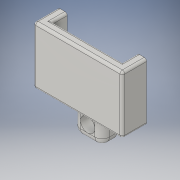
# Autodesk Inventor part: soporte esp1
Saved by Autodesk Inventor 2016 (Build 200138000, 138)
## iProperties
Created: 2017-03-11
Part Number: soporte esp1
Material: Generic
Document SubType Name: Modeling
Designer: jorge
Density: 1 g/cm^3
Appearance: White
Author: jorge
Autodesk Inventor part; units mm, degrees
ref_plane "YZ Plane" through (0, 0, 0) normal (1, 0, 0) x (0, 1, 0)
ref_plane "XZ Plane" through (0, 0, 0) normal (0, 1, 0) x (-1, 0, 0)
sketch "Sketch1" plane through (0, 0, 0) normal (0, 0, 1) x (1, 0, 0)
  line L0 (-32.1046, 28.3811) -> (-17.6046, 28.3811) projected
  line L1 (-32.1046, 3.3811) -> (-32.1046, 28.3811) projected
  line L2 (-17.6046, 3.3811) -> (-32.1046, 3.3811) projected
  line L3 (-17.6046, 28.3811) -> (-17.6046, 3.3811) projected
  circle A0 centre (-21.0446, 24.002) radius 0.51 projected
  circle A1 centre (-21.0446, 26.542) radius 0.51 projected
  circle A2 centre (-23.5846, 26.542) radius 0.51 projected
  circle A3 centre (-23.5846, 24.002) radius 0.51 projected
  circle A4 centre (-26.1246, 26.542) radius 0.51 projected
  circle A5 centre (-26.1246, 24.002) radius 0.51 projected
  circle A6 centre (-28.6646, 26.542) radius 0.51 projected
  circle A7 centre (-28.6646, 24.002) radius 0.51 projected
  line L4 (-17.6046, 3.3811) -> (-17.6046, 13.3811)
  line L5 (-17.6046, 13.3811) -> (-15.6046, 13.3811)
  line L6 (-15.6046, 13.3811) -> (-15.6046, 1.3811)
  line L7 (-15.6046, 1.3811) -> (-32.1046, 1.3811)
  line L8 (-32.1046, 1.3811) -> (-34.1046, 1.3811)
  line L9 (-34.1046, 1.3811) -> (-34.1046, 13.3811)
  line L10 (-34.1046, 13.3811) -> (-32.1046, 13.3811)
  point P0 (0, 0)
  dimension "d0" = 10
  dimension "d1" = 2
  dimension "d2" = 90
  dimension "d3" = 12
  dimension "d4" = 90
  dimension "d5" = 2
  dimension "d6" = 12
  constraints: 14 end point, 5 point on line, 2 perpendicular
  measures "d0" distance of L2.start L4.end
  measures "d1" distance of L4.end L5.end
  measures "d2" angle of L4 L5
  measures "d3" distance of L5.end L6.end
  measures "d4" angle of L6 L7
  measures "d5" distance of L7.end L8.end
  measures "d6" distance of L8.end L9.end
ref_plane "Work Plane1" through (-32.1046, 3.3811, 3.05) normal (0, 0, 1) x (1, 0, 0)
extrude "Extrusion1" add sketch "Sketch1" along normal up to surface (3.05 mm away) contours L1 L2 L3 L5 L6 L7 L8 L9 L10
sketch "Sketch2" plane through (-34.1046, 1.3811, 3.05) normal (0, 0, 1) x (1, 0, 0)
  line L0 (16.5, 12) -> (18.5, 12) projected
  line L1 (18.5, 12) -> (0, 12)
  line L2 (0, 12) -> (0, 0)
  line L3 (0, 0) -> (18.5, 0)
  line L4 (18.5, 0) -> (18.5, 12)
  point P0 (34.1046, -1.3811)
  constraints: 8 end point, 2 parallel, 1 horizontal, 1 perpendicular
extrude "Extrusion2" add sketch "Sketch2" along normal blind 2
sketch "Sketch3" plane through (-34.1046, 1.3811, 0) normal (0, -1, 0) x (1, 0, 0)
  line L0 (16.5, 0) -> (2, 0) projected
  line L1 (9.25, 0) -> (6.25, 0)
  line L2 (6.25, 0) -> (6.25, 3)
  line L3 (6.25, 3) -> (9.25, 3)
  line L4 (9.25, 3) -> (9.25, 0)
  line L5 (9.25, 3) -> (12.25, 3)
  line L6 (12.25, 3) -> (12.25, 0)
  line L7 (12.25, 0) -> (9.25, 0)
  line L8 (9.25, 0) -> (9.25, 3)
  point P0 (34.1046, 0)
  dimension "d11" = 3
  dimension "d12" = 3
  dimension "d13" = 3
  constraints: 16 end point, 4 parallel, 2 horizontal, 2 perpendicular, 1 midpoint, 1 point on line
  measures "d11" distance of L2.end L3.end
  measures "d12" distance of L1.end L2.end
  measures "d13" distance of L6.end L7.end
extrude "Extrusion3" add sketch "Sketch3" along normal blind 6
fillet "Fillet1" radius 1.5 8 edges at (-27.8546, -4.6189, 1.5) (-21.8546, -4.6189, 1.5) (-24.8546, 1.3811, 3) (-27.8546, 1.3811, 1.5) (-21.8546, 1.3811, 1.5) (-27.8546, -1.6189, 3) (-21.8546, -1.6189, 3) (-24.8546, -4.6189, 3)
sketch "Sketch4" plane through (-26.3546, -3.1189, 3) normal (0, 0, 1) x (1, 0, 0)
  line L0 (0, 3) -> (3, 3) projected
  line L1 (3, 3) -> (3, 0) projected
  circle A0 centre (1.5, 1.5) radius 1.5
  point P0 (26.3546, 3.1189)
  dimension "d17" = 3
  constraints: 1 centre point
  measures "d17" diameter of A0
extrude "Extrusion4" cut sketch "Sketch4" against normal blind 6 contours A0
fillet "Fillet2" radius 0.5 11 edges at (-15.6046, 1.3811, 2.525) (-34.1046, 1.3811, 2.525) (-24.8546, 1.3811, 5.05) (-34.1046, 13.3811, 2.525) (-24.8546, 13.3811, 5.05) (-15.6046, 13.3811, 2.525) (-24.8546, 13.3811, 3.05) (-17.6046, 13.3811, 1.525) (-32.1046, 13.3811, 1.525) (-34.1046, 7.3811, 5.05) (-15.6046, 7.3811, 5.05)
body "Solid1"
